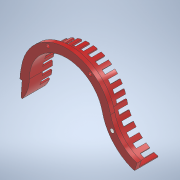
# Autodesk Inventor part: Intake Mustache
Saved by Autodesk Inventor 2022 (Build 260153000, 153)
## iProperties
Created: 2022-11-16
Part Number: Intake Mustache
Material: Generic
Document SubType Name: Modeling
Designer: matt
Density: 1 g/cm^3
Appearance: Default
Author: matt
Autodesk Inventor part; units mm, degrees
ref_plane "YZ Plane" through (0, 0, 0) normal (1, 0, 0) x (0, 1, 0)
sketch "Sketch1" plane through (0, 0, 0) normal (0, 0, 1) x (1, 0, 0)
  arc A0 (154.526, 70.2948) -> (52.5651, 41.6649) centre (107.5651, 41.6649) ccw
  line L0 (54.9684, 41.6649) -> (150.0445, 41.6649) construction
  line L1 (107.5651, 41.6649) -> (52.5651, 41.6649) construction
  line L2 (107.5651, 41.6649) -> (54.9602, 48.1239) construction
  line L3 (107.5651, 41.6649) -> (155.1965, 69.1649) construction
  arc A1 (54.9602, 48.1239) -> (54.5651, 41.6649) centre (107.5651, 41.6649) ccw
  line L4 (54.9602, 48.1239) -> (52.9763, 48.3772)
  line L5 (54.5651, 41.6649) -> (52.5651, 41.6649)
  arc A2 (152.8135, 69.2617) -> (54.5651, 41.6649) centre (107.5651, 41.6649) ccw
  arc A3 (170.9924, 55.8769) -> (43.6187, 53.3205) centre (107.5651, 41.6649) ccw
  line L6 (152.8135, 69.2617) -> (163.0885, 75.4607)
  circle A4 centre (81.2206, 96.1278) radius 2.8
  circle A5 centre (141.5591, 91.7114) radius 2.8
  arc A6 (161.2344, 53.6904) -> (52.5672, 42.1363) centre (107.5651, 41.6649) ccw
  line L7 (81.7174, 303.5602) -> (65.1074, 76.6268)
  line L8 (67.2133, 92.623) -> (66.1308, 77.8339)
  arc A7 (43.2754, 13.9907) -> (52.5672, 42.1363) centre (4.0333, 42.5523) ccw
  arc A8 (161.2344, 53.6904) -> (200.7542, 6.966) centre (225.6911, 68.1331) ccw
  line L9 (39.6637, 15.3137) -> (60.8975, 305.4174)
  arc A9 (39.6637, 15.3137) -> (43.2754, 13.9907) centre (41.6584, 15.1677) ccw
  arc A10 (200.7542, 6.966) -> (206.8445, 5.5395) centre (208.3045, 25.4861) ccw
  line L10 (209.3894, 5.3532) -> (206.8445, 5.5395)
  line L11 (230.4439, 293.0077) -> (209.3894, 5.3532)
  line L12 (232.4386, 292.8617) -> (211.2381, 3.2125)
  line L13 (211.2381, 3.2125) -> (206.6985, 3.5448)
  arc A11 (199.9991, 5.114) -> (206.6985, 3.5448) centre (208.3045, 25.4861) ccw
  arc A12 (159.2828, 53.2531) -> (199.9991, 5.114) centre (225.6911, 68.1331) ccw
  arc A13 (54.5651, 41.6649) -> (159.2828, 53.2531) centre (107.5651, 41.6649) ccw construction
  arc A14 (44.8925, 12.8138) -> (54.5671, 42.1192) centre (4.0333, 42.5523) ccw
  arc A15 (37.6691, 15.4597) -> (44.8925, 12.8138) centre (41.6584, 15.1677) ccw
  line L14 (37.6691, 15.4597) -> (58.9028, 305.5634)
  line L15 (43.6187, 53.3205) -> (41.6584, 42.5656)
  line L16 (4.0333, 42.5523) -> (54.5651, 41.6649) construction
  line L17 (4.0333, 42.5523) -> (52.2065, 36.6321) construction
  line L18 (4.0333, 42.5523) -> (54.5689, 42.5523) construction
  line L19 (52.2065, 36.6321) -> (54.1916, 36.3882)
  line L20 (51.0217, 30.3949) -> (52.9579, 29.894)
  line L21 (49.0328, 24.3657) -> (50.8871, 23.6163)
  line L22 (46.274, 18.6477) -> (48.0146, 17.6627)
  line L23 (42.7924, 13.3387) -> (44.3896, 12.1349)
  line L24 (42.6615, 13.4374) -> (44.3234, 12.1848) construction
  line L25 (42.6615, 13.4374) -> (44.3234, 12.1848)
  line L26 (39.1312, 35.4357) -> (41.1258, 35.2897)
  line L27 (41.1258, 35.2897) -> (40.1285, 21.6637)
  line L28 (40.1285, 21.6637) -> (43.2469, 21.4355)
  line L29 (42.6615, 13.4374) -> (44.2442, 35.0614)
  line L30 (44.2442, 35.0614) -> (41.1258, 35.2897)
  line L31 (107.5651, 41.6649) -> (159.2828, 53.2531) construction
  line L32 (55.911, 53.5329) -> (53.9639, 53.9901)
  line L33 (57.4164, 58.8144) -> (55.5271, 59.4706)
  line L34 (59.4603, 63.9117) -> (57.649, 64.76)
  line L35 (62.0207, 68.7702) -> (60.3069, 69.8013)
  line L36 (65.07, 73.3377) -> (63.4722, 74.5406)
  line L37 (68.5757, 77.5651) -> (67.1109, 78.9269)
  line L38 (72.5, 81.407) -> (71.184, 82.9131)
  line L39 (76.8008, 84.8222) -> (75.6477, 86.4564)
  line L40 (81.4319, 87.774) -> (80.4541, 89.5187)
  line L41 (86.3436, 90.2308) -> (85.5516, 92.0673)
  line L42 (91.4832, 92.1661) -> (90.8855, 94.0747)
  line L43 (96.7954, 93.5591) -> (96.3985, 95.5193)
  line L44 (102.2233, 94.395) -> (102.0313, 96.3858)
  line L45 (107.7086, 94.6647) -> (107.7236, 96.6646)
  line L46 (113.1923, 94.3653) -> (113.4142, 96.353)
  line L47 (118.6155, 93.5001) -> (119.0419, 95.4541)
  line L48 (123.9201, 92.0783) -> (124.5465, 93.9777)
  line L49 (129.0492, 90.1152) -> (129.8687, 91.9396)
  line L50 (133.9475, 87.6319) -> (134.9514, 89.3617)
  line L51 (138.5626, 84.6551) -> (139.7401, 86.2717)
  line L52 (142.8448, 81.2166) -> (144.1833, 82.7028)
  line L53 (146.7483, 77.3535) -> (148.2334, 78.6932)
  line L54 (150.231, 73.1072) -> (151.8468, 74.286)
  line L55 (153.2556, 68.5233) -> (154.9847, 69.5286)
  line L56 (155.7897, 63.651) -> (157.6135, 64.472)
  line L57 (157.8059, 58.5427) -> (159.7049, 59.1705)
  line L58 (159.2828, 53.2531) -> (161.2365, 53.681)
  arc A16 (159.2828, 53.2531) -> (54.5671, 42.1192) centre (107.5651, 41.6649) ccw
  arc A17 (170.9924, 55.8769) -> (212.0111, 13.773) centre (225.6911, 68.1331) ccw
  arc A18 (220.0721, 123.9057) -> (218.0491, 123.6647) centre (225.6911, 68.1331) ccw
  line L59 (225.6911, 68.1331) -> (159.2828, 53.2531) construction
  line L60 (225.6911, 68.1331) -> (162.7384, 48.1276) construction
  line L61 (162.7384, 48.1276) -> (160.8323, 47.5219)
  line L62 (225.6911, 68.1331) -> (208.9559, 14.6346) construction
  line L63 (206.1312, 5.6045) -> (205.5237, 3.6625)
  line L64 (208.9559, 14.6346) -> (206.1312, 5.6045)
  line L65 (164.9457, 42.186) -> (163.1064, 41.4003)
  line L66 (167.7122, 36.4832) -> (165.9568, 35.5249)
  line L67 (171.0127, 31.0719) -> (169.3571, 29.9498)
  line L68 (174.8166, 26.0018) -> (173.2762, 24.7262)
  line L69 (179.0889, 21.3197) -> (177.6779, 19.9023)
  line L70 (183.7903, 17.0686) -> (182.5216, 15.5225)
  line L71 (188.8775, 13.2877) -> (187.7629, 11.6271)
  line L72 (194.3037, 10.0118) -> (193.3534, 8.252)
  line L73 (200.0189, 7.271) -> (199.2416, 5.4282)
  line L74 (205.9704, 5.0906) -> (205.3734, 3.1818)
  line L75 (107.5651, 41.6649) -> (81.2206, 96.1278) construction
  line L76 (107.5651, 41.6649) -> (141.5591, 91.7114) construction
  line L77 (107.5651, 41.6649) -> (194.2194, 35.3223) construction
  circle A19 centre (173.2554, 36.8568) radius 2.8
  point P0 (0, 0)
  point P1 (54.9602, 48.1239)
  point P2 (154.526, 70.2948)
  point P3 (66.2194, 91.8199)
  point P4 (66.1308, 77.8339)
  point P5 (54.5611, 41.6649)
  point P6 (52.5672, 42.1363)
  point P7 (54.5671, 42.1192)
  point P8 (154.526, 70.2948)
  point P9 (152.8135, 69.2617)
  point P10 (152.8135, 69.2617)
  point P11 (154.526, 70.2948)
  point P12 (210.0447, 14.3061)
  point P13 (159.2828, 53.2531)
  dimension "d0" = 55
  dimension "d3" = 0
  dimension "d5" = 2
  dimension "d10" = 7
  dimension "d15" = 5.6
  dimension "d16" = 5.6
  dimension "d19" = 65
  dimension "d21" = 2
  dimension "d22" = 50.5357
  dimension "d24" = 6
  dimension "d27" = 30
  dimension "d35" = 160.37
  dimension "d38" = 160.37
  dimension "d40" = 68.055
  dimension "d42" = 5
  dimension "d44" = 55
  dimension "d51" = 55
  dimension "d53" = 60
  dimension "d54" = 60
  dimension "d55" = 5.6
  dimension "d56" = 2.2
  constraints: 156 end point, 45 point on circle, 18 centre point, 12 point on line, 3 parallel, 2 coincident, 2 horizontal, 2 perpendicular, 1 collinear, 1 tangent, 168 other
  measures "d3" distance between parallel lines of L0 L1
  measures "d10" angle of L2 L1
  measures "d15" diameter of A4
  measures "d16" diameter of A5
  measures "d19" radius of A3
  measures "d21" radial gap between concentric circles of A7 A14
  measures "d22" radius of A14
  measures "d24" angle of L17 L16
  measures "d35" angle of L31 L2
  measures "d40" radius of A12
  measures "d42" angle of L60 L59
  measures "d44" angle of L62 L60
  measures "d53" angle of L76 L75
  measures "d54" angle of L77 L76
  measures "d55" diameter of A19
extrude "Extrusion1" add sketch "Sketch1" against normal blind 14 contours L6 A2 L54 A0 | A6 L55 A16 L6 | L53 A2 L52 A0 | A6 L57 A16 L56 | A0 L37 A2 L36 | L51 A2 L50 A0 | L63 A11 A12 L73 A8 A10 | L58 A8 L61 A12 | A0 L39 A2 L38 | L49 A2 L48 A0 | L35 A2 L34 A0 | L65 A8 L66 A12 | L72 A12 L71 A8 | A0 L41 A2 L40 | L47 A2 L46 A0 | L33 A2 L32 A0 | L67 A8 L68 A12 | L70 A12 L69 A8 | A9 A7 L22 A14 A15 L23 L25 | A0 L43 A2 L42 | L45 A2 L44 A0 | L4 A1 A14 L5 A0 | A7 L21 A14 L22 | L19 A14 L20 A7 | A1 L5 A14
extrude "Extrusion2" add sketch "Sketch1" along normal blind 19 contours L6 A2 L54 A0 | A6 L55 A16 L6 | L54 A2 L53 A0 | A6 L56 A16 L55 | L53 A2 L52 A0 | A6 L57 A16 L56 | L52 A2 L51 A0 | A0 L37 A2 L36 | A6 A8 L58 A16 L57 | L51 A2 L50 A0 | L63 A11 A12 L73 A8 A10 | A0 L38 A2 L37 | L50 A2 L49 A0 | L58 A8 L61 A12 | L36 A2 L35 A0 | A0 L39 A2 L38 | L49 A2 L48 A0 | L61 A8 L65 A12 | L73 A12 L72 A8 | L35 A2 L34 A0 | A0 L40 A2 L39 | L48 A2 L47 A0 | L65 A8 L66 A12 | L72 A12 L71 A8 | L34 A2 L33 A0 | A0 L41 A2 L40 | L47 A2 L46 A0 | L66 A8 L67 A12 | L71 A12 L70 A8 | L33 A2 L32 A0 | A0 L42 A2 L41 | L46 A2 L45 A0 | L67 A8 L68 A12 | L70 A12 L69 A8 | A9 A7 L22 A14 A15 L23 L25 | L32 A2 L4 A0 | A0 L43 A2 L42 | L45 A2 L44 A0 | L68 A8 L69 A12 | L4 A1 A14 L5 A0 | A0 L44 A2 L43 | A7 L21 A14 L22 | A0 L5 A14 L19 A7 | A7 L20 A14 L21 | L19 A14 L20 A7 | A1 L5 A14
ref_plane "Work Plane1" through (39.3025, 55.1816, 16.3) normal (0, 0, 1) x (0.9973, -0.073, 0)
ref_plane "Work Plane2" through (39.5177, 0.9093, 13) normal (0, 0, 1) x (0.9973, -0.073, 0)
extrude "Extrusion3" add sketch "Sketch1" against normal up to surface (6 mm away) from surface at 19 contours A0 L8 A3 L6 | L6 A3 A17 L64 A10 A8 A6
extrude "Extrusion5" add sketch "Sketch1" against normal blind 2.7 from surface at 19 contours L8 A0 L7 A3 | L7 A0 A7 A9 L29 L30 L9 L15 A3
equation "\"d38\" = d35"
body "Solid1"
